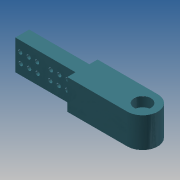
# Autodesk Inventor part: driven arm2_2
Saved by Autodesk Inventor 2013 (Build 170138000, 138)
## iProperties
Created: 2017-03-30
Part Number: driven arm2_2
Material: Generic
Document SubType Name: Modeling
Designer: employee
Density: 1 g/cm^3
Author: employee
Autodesk Inventor part; units mm, degrees
ref_plane "YZ Plane" through (0, 0, 0) normal (1, 0, 0) x (0, 1, 0)
ref_plane "XZ Plane" through (0, 0, 0) normal (0, 1, 0) x (-1, 0, 0)
ref_plane "XY Plane" through (0, 0, 0) normal (0, 0, 1) x (1, 0, 0)
sketch "Sketch1" plane through (0, 0, 0) normal (0, 0, 1) x (1, 0, 0)
  line L0 (0, 12.6) -> (153, 12.6)
  arc A0 (153, -12.6) -> (153, 12.6) centre (153, 0) ccw
  line L1 (153, -12.6) -> (0, -12.6)
  arc A1 (0, 12.6) -> (0, -12.6) centre (0, 0) ccw
  circle A2 centre (0, 0) radius 7.5
  circle A3 centre (153, 0) radius 4.25
  dimension "d0" = 153
  dimension "d2" = 12.6
  dimension "d3" = 15
  dimension "d4" = 8.5
  constraints: 4 centre point, 4 end point, 4 point on circle, 4 tangent, 3 coincident, 1 horizontal, 1 parallel
  measures "d0" distance of L0.start L0.end
  measures "d2" radius of A1
  measures "d3" diameter of A2
  measures "d4" diameter of A3
extrude "Extrusion1" add sketch "Sketch1" along normal blind 25
sketch "Sketch2" plane through (0, 0, 25) normal (0, 0, 1) x (1, 0, 0)
  circle A0 centre (0, 0) radius 7.5 projected
  arc A1 (0, 12.6) -> (0, -12.6) centre (0, 0) ccw projected
  circle A2 centre (0, 0) radius 11
  dimension "d7" = 22
  constraints: 1 centre point, 1 coincident
  measures "d7" diameter of A2
extrude "Extrusion2" cut sketch "Sketch2" against normal blind 7
sketch "Sketch4" plane through (0, 0, 25) normal (0, 0, 1) x (1, 0, 0)
  circle A0 centre (0, 0) radius 11 projected
  circle A1 centre (20, 0) radius 1.75
  circle A2 centre (40, 0) radius 1.75
  dimension "d16" = 20
  dimension "d17" = 40
  dimension "d23" = 3.5
  constraints: 2 centre point, 2 horizontal alignment, 1 equal radius
  measures "d16" distance of A1.centre A0.centre
  measures "d17" distance of A2.centre A0.centre
  measures "d23" diameter of A1
extrude "Extrusion3" cut sketch "Sketch4" against normal through all contours A1 | A2
sketch "Sketch5" plane through (0, 0, 25) normal (0, 0, 1) x (1, 0, 0)
  circle A0 centre (20, 0) radius 1.75 projected
  circle A1 centre (40, 0) radius 1.75 projected
  circle A2 centre (40, 0) radius 3
  circle A3 centre (20, 0) radius 3
  dimension "d28" = 6
  constraints: 2 centre point, 2 coincident, 1 equal radius
  measures "d28" diameter of A3
extrude "Extrusion4" cut sketch "Sketch5" against normal blind 3
sketch "Sketch6" plane through (0, 0, 25) normal (0, 0, 1) x (1, 0, 0)
  line L0 (153, 12.6) -> (0, 12.6) projected
  arc A0 (0, 12.6) -> (0, -12.6) centre (0, 0) ccw projected
  line L1 (0, -12.6) -> (153, -12.6) projected
  arc A1 (12.1445, 12.6) -> (12.1445, -12.6) centre (0, 0) ccw
  dimension "d24" = 35
  constraints: 2 point on circle, 2 point on line, 1 centre point, 1 coincident
  measures "d24" diameter of A1
extrude "Extrusion5" add sketch "Sketch6" against normal up to surface (25 mm away)
sketch "Sketch7" plane through (0, 0, 25) normal (0, 0, 1) x (1, 0, 0)
  circle A0 centre (153, 0) radius 4.25 projected
  arc A1 (153, -12.6) -> (153, 12.6) centre (153, 0) ccw projected
  circle A2 centre (153, 0) radius 7
  dimension "d30" = 14
  constraints: 1 centre point, 1 coincident
  measures "d30" diameter of A2
extrude "Extrusion6" cut sketch "Sketch7" against normal blind 8
fillet "Fillet1" radius 3.5 1 edges at (-7.5, 0, 18)
sketch "Sketch8" plane through (0, 0, 25) normal (0, 0, 1) x (1, 0, 0)
  circle A0 centre (153, 0) radius 7 projected
  line L0 (153, 12.6) -> (12.1445, 12.6) projected
  arc A1 (12.1445, 12.6) -> (12.1445, -12.6) centre (0, 0) ccw projected
  line L1 (12.1445, -12.6) -> (153, -12.6) projected
  line L2 (103, 12.6) -> (103, 5.75)
  line L3 (103, 5.75) -> (53, 5.75)
  line L4 (53, 5.75) -> (53, -5.75)
  line L5 (53, -5.75) -> (103, -5.75)
  line L6 (103, -5.75) -> (103, -12.6)
  dimension "d35" = 50
  dimension "d36" = 50
  dimension "d37" = 11.5
  constraints: 10 end point, 3 perpendicular, 2 equal length, 2 parallel, 2 point on line
  measures "d35" distance from line of L2 A0.centre
  measures "d36" distance between parallel lines of L4 L2
  measures "d37" distance between parallel lines of L3 L5
extrude "Extrusion7" cut sketch "Sketch8" against normal through all contours L2 L3 L4 L5 L6 L1 A1 L0
sketch "Sketch9" plane through (53, -5.75, 25) normal (0, -1, 0) x (1, 0, 0)
  line L0 (0, 0) -> (0, -25) projected
  line L1 (4.5, -8.5) -> (12.5, -8.5) construction
  line L2 (12.5, -8.5) -> (12.5, -16.5) construction
  line L3 (12.5, -16.5) -> (4.5, -16.5) construction
  line L4 (4.5, -16.5) -> (4.5, -8.5) construction
  line L5 (12.5, -16.5) -> (20.5, -16.5) construction
  line L6 (20.5, -16.5) -> (20.5, -8.5) construction
  line L7 (20.5, -8.5) -> (12.5, -8.5) construction
  line L8 (12.5, -8.5) -> (12.5, -16.5) construction
  circle A0 centre (4.5, -16.5) radius 1.75
  circle A1 centre (4, -8.5) radius 1.75
  circle A2 centre (11.5, -16.5) radius 1.75
  circle A3 centre (11, -8.5) radius 1.75
  circle A4 centre (18.5, -16.5) radius 1.75
  circle A5 centre (18, -8.5) radius 1.75
  line L9 (29.5, -8.5) -> (37.5, -8.5) construction
  line L10 (37.5, -8.5) -> (37.5, -16.5) construction
  line L11 (37.5, -16.5) -> (29.5, -16.5) construction
  line L12 (29.5, -16.5) -> (29.5, -8.5) construction
  line L13 (37.5, -16.5) -> (45.5, -16.5) construction
  line L14 (45.5, -16.5) -> (45.5, -8.5) construction
  line L15 (45.5, -8.5) -> (37.5, -8.5) construction
  line L16 (37.5, -8.5) -> (37.5, -16.5) construction
  circle A6 centre (29.5, -8.5) radius 1.75
  circle A7 centre (29, -16.5) radius 1.75
  circle A8 centre (36.5, -8.5) radius 1.75
  circle A9 centre (36, -16.5) radius 1.75
  circle A10 centre (43.5, -8.5) radius 1.75
  circle A11 centre (43, -16.5) radius 1.75
  point P0 (-53, -25)
  point P1 (0, -12.5)
  point P2 (12.5, -12.5)
  point P3 (12.5, -12.5)
  point P4 (37.5, -12.5)
  dimension "d40" = 12.5
  dimension "d41" = 8
  dimension "d42" = 0.5
  dimension "d43" = 1
  dimension "d44" = 1.5
  dimension "d45" = 2
  dimension "d46" = 2.5
  dimension "d47" = 3.5
  dimension "d48" = 25
  dimension "d49" = 0.5
  dimension "d50" = 1
  dimension "d51" = 1.5
  dimension "d52" = 2
  dimension "d53" = 2.5
  constraints: 32 end point, 12 centre point, 11 equal radius, 8 parallel, 8 point on line, 5 equal length, 4 horizontal, 4 horizontal alignment, 4 midpoint, 4 perpendicular, 2 coincident
  measures "d40" distance from line of L1.end L0
  measures "d41" distance of L3.end L1.start
  measures "d42" distance of A1.centre L1.start
  measures "d43" distance of A2.centre L2.end
  measures "d44" distance from line of A3.centre L2
  measures "d45" distance from line of A4.centre L6
  measures "d46" distance from line of A5.centre L6
  measures "d47" diameter of A1
  measures "d48" distance from line of L2 point (37.5, -12.5)
  measures "d49" distance of A7.centre L11.end
  measures "d50" distance from line of A8.centre L16
  measures "d51" distance from line of A9.centre L10
  measures "d52" distance from line of A10.centre L14
  measures "d53" distance from line of A11.centre L14
extrude "Extrusion8" cut sketch "Sketch9" against normal through all
body "Solid1"
